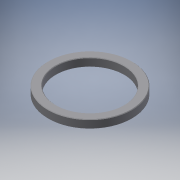
# Autodesk Inventor part: 零件6
Saved by Autodesk Inventor 2018 (Build 220112000, 112)
## iProperties
Created: 2017-07-24
Part Number: 零件6
Material: 一般
Document SubType Name: Modeling
Designer: Alex
Density: 1 g/cm^3
Appearance: 預設
Author: Alex
Autodesk Inventor part; units mm, degrees
ref_plane "YZ Plane" through (0, 0, 0) normal (1, 0, 0) x (0, 1, 0)
ref_plane "XZ Plane" through (0, 0, 0) normal (0, 1, 0) x (-1, 0, 0)
ref_plane "XY Plane" through (0, 0, 0) normal (0, 0, 1) x (1, 0, 0)
sketch "草圖1" plane through (0, 0, 0) normal (0, 0, 1) x (1, 0, 0)
  circle A0 centre (0, 0) radius 12.525
  circle A1 centre (0, 0) radius 15.525
  dimension "d0" = 25.05
  dimension "d11" = 31.05
  dimension "d12" = 3
  constraints: 2 centre point, 2 coincident
  measures "d0" diameter of A0
  measures "d11" diameter of A1
  measures "d12" radial gap between concentric circles of A0 A1
extrude "擠出1" add sketch "草圖1" along normal blind 3.05
chamfer "倒角1" distance 0.2 angle 45 4 edges at (-15.525, 0, 3.05) (-15.525, 0, 0) (-12.525, 0, 0) (-12.525, 0, 3.05)
